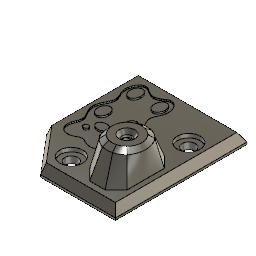
filament_sensor_cover_pc4-m10 (Autodesk Fusion 360 archive; units mm, degrees)
design "filament_sensor_cover"
Autodesk Fusion 360 part; units mm, degrees
sketch "base" plane through (0, 0, 0) normal (0, 0, 1) x (1, 0, 0)
  line L0 (0, 0) -> (27.1, 0)
  line L1 (27.1, 0) -> (27.1, 33.5)
  line L2 (27.1, 33.5) -> (0, 33.5)
  line L3 (0, 33.5) -> (0, 0)
  circle A0 centre (22.25, 23.5) radius 1.65
  circle A1 centre (20.05, 10) radius 2.2
  circle A2 centre (10.4, 5.5) radius 1.65
  circle A3 centre (20.05, 10) radius 1.3
  circle A4 centre (20.05, 10) radius 4.75
  line L4 (0, 9.5936) -> (8.05, 0)
  line L5 (24.8, 14.75) -> (24.8, 5.25)
  line L6 (24.8, 5.25) -> (22.0175, 2.4675)
  line L7 (22.0175, 2.4675) -> (18.0825, 2.4675)
  line L8 (18.0825, 2.4675) -> (15.3, 5.25)
  line L9 (15.3, 5.25) -> (15.3, 14.75)
  line L10 (24.8, 14.75) -> (22.0175, 17.5325)
  line L11 (22.0175, 17.5325) -> (18.0825, 17.5325)
  line L12 (18.0825, 17.5325) -> (15.3, 14.75)
  circle A5 centre (10.4, 5.5) radius 2.9
  circle A6 centre (22.25, 23.5) radius 2.9
  dimension "d4" = 3.3
  dimension "d5" = 3.3
  dimension "d6" = 4.4
  dimension "d7" = 2.6
  dimension "d11" = 2.2
  dimension "d15" = 9.65
  dimension "d21" = 9.5
  dimension "d78" = 10
  dimension "d85" = 20.05
  dimension "d94" = 7.05
  dimension "d139" = 13.5
  dimension "d141" = 4.5
  dimension "d142" = 40
  dimension "d151" = 45
  dimension "d152" = 45
  dimension "d153" = 9.5
  dimension "d154" = 45
  dimension "d155" = 45
  dimension "d159" = 5.8
  dimension "d160" = 5.8
  dimension "d163" = 23.5
  dimension "d166" = 12
  measures "d4" diameter of A0
  measures "d5" diameter of A2
  measures "d6" diameter of A1
  measures "d7" diameter of A3
  measures "d11" distance of L0.start
  measures "d21" diameter of A4
  measures "d85" distance of L0.start
  measures "d139" distance of L0.start
  measures "d142" angle of L3 L4
  measures "d151" angle of L7 L8
  measures "d152" angle of L6 L7
  measures "d154" angle of L11 L12
  measures "d155" angle of L10 L11
  measures "d159" diameter of A5
  measures "d160" diameter of A6
extrude "Extrude1" add sketch "base" against normal blind 3 contours L0 L1 L2 L3 L4 | A4 L5 L6 L7 L8 L9 | A4 L5 L9 L10 L11 L12 | A5 | A6
extrude "Extrude3" add sketch "base" along normal blind 7.5 and the other way up to surface (3 mm away) contours A1 | A3 | A4
loft "Loft1" add profiles "base" section 1 contours A1 | A3 | A4 | A4 L5 L6 L7 L8 L9 | A4 L5 L9 L10 L11 L12 section 2 face at (21.2351, 11.0499, 7.5)
extrude "Extrude12" cut sketch "base" along normal mid plane 20 contours A1 | A3
extrude "Extrude4" add sketch "base" against normal blind 2 from surface at 7.5 contours A1
extrude "Extrude16" cut sketch "base" against normal blind 1 contours A5 | A6
chamfer "Chamfer1" distance 1 angle 45 8 edges at (20.05, 5.25, 7.5) (17.688, 5.8789, 7.5) (24.8, 10, 7.5) (22.4315, 14.1099, 7.5) (20.0725, 14.7499, 7.5) (17.688, 14.1211, 7.5) (15.3, 10, 7.5) (22.412, 5.8789, 7.5)
chamfer "Chamfer2" distance 1 distance2 0.7 1 edges at (18.838, 9.5299, 7.5) measured on face at (21.3435, 9.8706, 6.8333)
chamfer "Chamfer4" distance 1 distance2 2.4 4 edges at (4.025, 4.7968, 0) (0, 21.5468, 0) (27.1, 16.75, 0) (17.575, 0, 0) measured on face at (5.1, 19.2812, 0) measured on face at (5.1, 19.2812, 0) measured on face at (5.1, 19.2812, 0) measured on face at (5.1, 19.2812, 0)
chamfer "Chamfer15" distance 1.6 distance2 2.4 1 edges at (13.55, 33.5, 0) measured on face at (5.7667, 19.4025, 0)
chamfer "Chamfer22" distance 0.3 angle 45 2 edges at (8.8617, 4.9033, -3) (20.7117, 22.9033, -3)
sketch "in_air_hole" plane through (0, 0, 5.5) normal (0, 0, -1) x (1, 0, 0)
  line L0 (18.2752, -8.7) -> (21.8248, -8.7)
  line L1 (18.2752, -11.3) -> (21.8248, -11.3)
  line L2 (21.35, -8.7) -> (21.35, -11.3)
  line L3 (18.75, -8.7) -> (18.75, -11.3)
  circle A0 centre (20.05, -10) radius 1.3
  circle A1 centre (20.05, -10) radius 2.2
extrude "Extrude10" cut sketch "in_air_hole" against normal blind 0.2 contours L0 L1 L3 A1 | L0 L1 L2 A1
extrude "Extrude11" cut sketch "in_air_hole" against normal blind 0.4 contours L0 L3 A0 | L0 L2 A0 | L1 L3 A0 | L1 L2 A0
sketch "Sketch12" plane through (0, 0, -3) normal (0, 0, -1) x (1, 0, 0)
  circle A0 centre (20.05, -10) radius 2.2
  line L0 (8.05, 0) -> (0, -9.5936)
  line L1 (0, -9.5936) -> (0, -33.5)
  line L2 (0, -33.5) -> (27.1, -33.5)
  line L3 (27.1, -33.5) -> (27.1, 0)
  line L4 (27.1, 0) -> (8.05, 0)
  circle A1 centre (20.05, -10) radius 2.2
  line L5 (0, -33.5) -> (27.1, -33.5)
  line L6 (23.85, -2.4) -> (16.55, -2.4)
  line L7 (16.55, -2.4) -> (16.55, -18.3)
  line L8 (16.55, -18.3) -> (23.85, -18.3)
  line L9 (23.85, -18.3) -> (23.85, -2.4)
  line L10 (16.55, -7.5) -> (23.85, -7.5)
  line L11 (16.55, -12.5) -> (23.85, -12.5)
  line L12 (22.55, -7.5) -> (22.55, -12.5)
  line L13 (17.55, -7.5) -> (17.55, -12.5)
  line L14 (6.25, -8.7) -> (9.35, -8.7)
  line L15 (9.35, -8.7) -> (9.35, -26.3)
  line L16 (9.35, -26.3) -> (6.25, -26.3)
  line L17 (6.25, -26.3) -> (6.25, -8.7)
  circle A2 centre (20.05, -10) radius 2.5
  circle A3 centre (10.4, -5.5) radius 1.95
  dimension "d239" = 3.8
  dimension "d240" = 7.6
  dimension "d241" = 3.5
  dimension "d242" = 8.3
  dimension "d249" = 3.1
  dimension "d251" = 17.6
  dimension "d252" = 10.7
  dimension "d254" = 0.3
  dimension "d259" = 3.2
  measures "d239" distance of L9
  measures "d240" distance of L6
  measures "d241" distance of L7
  measures "d242" distance of L8
  measures "d249" distance of L15 L17
  measures "d252" distance of L15
  measures "d254" distance of A0 A2
  measures "d259" distance of L14
extrude "Extrude17" cut sketch "Sketch12" against normal blind 1.4 contours L6 L7 L9 L10 | L9 L10 L11 L12 | L7 L10 L11 L13 | L7 L8 L9 L11 | L10 L12 A2 | L10 L13 A2 | L11 L12 A2 | A2 | L11 L13 A2 | L14 L15 L16 L17
extrude "Extrude19" cut sketch "Sketch12" against normal blind 0.2 from surface at -1.4 contours L9 L10 L11 L12 | L7 L10 L11 L13
extrude "Extrude20" cut sketch "Sketch12" against normal blind 0.4 from surface at -1.4 contours A0 A1 | L10 L12 A2 | L10 L13 A2 | L11 L12 A2 | A2 | L11 L13 A2
extrude "Extrude21" cut sketch "Sketch12" against normal blind 0.5 draft -45 from surface at -1.8 contours A0 A1 | A2
chamfer "Chamfer21" distance 0.5 angle 45 5 edges at (6.25, 17.5, -3) (9.35, 17.5, -3) (7.8, 8.7, -3) (23.85, 10.35, -3) (20.2, 2.4, -3)
sketch "logo" plane through (0, 0, 0) normal (0, 0, 1) x (-1, 0, 0)
  line L0 (-7.6627, -29.107) -> (-7.9745, -29.1444)
  line L1 (-7.9745, -29.1444) -> (-8.3459, -29.2538)
  line L2 (-8.3459, -29.2538) -> (-8.7523, -29.427)
  line L3 (-8.7523, -29.427) -> (-9.1647, -29.6489)
  line L4 (-9.1647, -29.6489) -> (-9.5618, -29.8965)
  line L5 (-9.5618, -29.8965) -> (-9.9376, -30.1385)
  line L6 (-9.9376, -30.1385) -> (-10.3005, -30.3388)
  line L7 (-10.3005, -30.3388) -> (-10.6648, -30.4618)
  line L8 (-10.6648, -30.4618) -> (-11.0429, -30.4781)
  line L9 (-11.0429, -30.4781) -> (-11.4365, -30.37)
  line L10 (-11.4365, -30.37) -> (-11.834, -30.1332)
  line L11 (-11.834, -30.1332) -> (-12.214, -29.7753)
  line L12 (-12.214, -29.7753) -> (-12.5496, -29.3123)
  line L13 (-12.5496, -29.3123) -> (-12.8133, -28.7661)
  line L14 (-12.8133, -28.7661) -> (-12.9814, -28.1613)
  line L15 (-12.9814, -28.1613) -> (-13.0387, -27.5233)
  line L16 (-13.0387, -27.5233) -> (-12.9808, -26.8757)
  line L17 (-12.9808, -26.8757) -> (-12.8192, -26.2395)
  line L18 (-12.8192, -26.2395) -> (-12.5836, -25.6303)
  line L19 (-12.5836, -25.6303) -> (-12.3262, -25.0573)
  line L20 (-12.3262, -25.0573) -> (-12.1178, -24.521)
  line L21 (-12.1178, -24.521) -> (-12.0118, -24.0146)
  line L22 (-12.0118, -24.0146) -> (-12.0257, -23.526)
  line L23 (-12.0257, -23.526) -> (-12.1502, -23.042)
  line L24 (-12.1502, -23.042) -> (-12.358, -22.5502)
  line L25 (-12.358, -22.5502) -> (-12.6136, -22.0431)
  line L26 (-12.6136, -22.0431) -> (-12.8804, -21.5194)
  line L27 (-12.8804, -21.5194) -> (-13.1248, -20.9829)
  line L28 (-13.1248, -20.9829) -> (-13.318, -20.4413)
  line L29 (-13.318, -20.4413) -> (-13.438, -19.9032)
  line L30 (-13.438, -19.9032) -> (-13.4715, -19.3767)
  line L31 (-13.4715, -19.3767) -> (-13.4161, -18.8673)
  line L32 (-13.4161, -18.8673) -> (-13.2803, -18.3767)
  line L33 (-13.2803, -18.3767) -> (-13.0813, -17.9044)
  line L34 (-13.0813, -17.9044) -> (-12.8431, -17.4481)
  line L35 (-12.8431, -17.4481) -> (-12.593, -17.005)
  line L36 (-12.593, -17.005) -> (-12.36, -16.5737)
  line L37 (-12.36, -16.5737) -> (-12.1707, -16.1535)
  line L38 (-12.1707, -16.1535) -> (-12.048, -15.7441)
  line L39 (-12.048, -15.7441) -> (-12.0061, -15.3438)
  line L40 (-12.0061, -15.3438) -> (-12.0482, -14.948)
  line L41 (-12.0482, -14.948) -> (-12.1635, -14.5478)
  line L42 (-12.1635, -14.5478) -> (-12.328, -14.1315)
  line L43 (-12.328, -14.1315) -> (-12.5094, -13.6882)
  line L44 (-12.5094, -13.6882) -> (-12.6717, -13.2115)
  line L45 (-12.6717, -13.2115) -> (-12.7802, -12.7035)
  line L46 (-12.7802, -12.7035) -> (-12.8062, -12.1779)
  line L47 (-12.8062, -12.1779) -> (-12.7291, -11.6578)
  line L48 (-12.7291, -11.6578) -> (-12.5377, -11.1715)
  line L49 (-12.5377, -11.1715) -> (-12.2318, -10.7487)
  line L50 (-12.2318, -10.7487) -> (-11.8228, -10.4149)
  line L51 (-11.8228, -10.4149) -> (-11.3348, -10.1886)
  line L52 (-11.3348, -10.1886) -> (-10.8008, -10.0778)
  line L53 (-10.8008, -10.0778) -> (-10.2568, -10.0804)
  line L54 (-10.2568, -10.0804) -> (-9.7352, -10.1825)
  line L55 (-9.7352, -10.1825) -> (-9.2581, -10.3582)
  line L56 (-9.2581, -10.3582) -> (-8.8319, -10.5692)
  line L57 (-8.8319, -10.5692) -> (-8.4472, -10.7692)
  line L58 (-8.4472, -10.7692) -> (-8.087, -10.9124)
  line L59 (-8.087, -10.9124) -> (-7.7345, -10.9646)
  line L60 (-7.6627, -29.107) -> (-7.3505, -29.1419)
  line L61 (-7.3505, -29.1419) -> (-6.9782, -29.2483)
  line L62 (-6.9782, -29.2483) -> (-6.5705, -29.4184)
  line L63 (-6.5705, -29.4184) -> (-6.1563, -29.637)
  line L64 (-6.1563, -29.637) -> (-5.7572, -29.8814)
  line L65 (-5.7572, -29.8814) -> (-5.3795, -30.1203)
  line L66 (-5.3795, -30.1203) -> (-5.0151, -30.3179)
  line L67 (-5.0151, -30.3179) -> (-4.6498, -30.4379)
  line L68 (-4.6498, -30.4379) -> (-4.2717, -30.4513)
  line L69 (-4.2717, -30.4513) -> (-3.8789, -30.34)
  line L70 (-3.8789, -30.34) -> (-3.4832, -30.1001)
  line L71 (-3.4832, -30.1001) -> (-3.1061, -29.7391)
  line L72 (-3.1061, -29.7391) -> (-2.7742, -29.2735)
  line L73 (-2.7742, -29.2735) -> (-2.5149, -28.7253)
  line L74 (-2.5149, -28.7253) -> (-2.3514, -28.1192)
  line L75 (-2.3514, -28.1192) -> (-2.2993, -27.4807)
  line L76 (-2.2993, -27.4807) -> (-2.3622, -26.8337)
  line L77 (-2.3622, -26.8337) -> (-2.5289, -26.1987)
  line L78 (-2.5289, -26.1987) -> (-2.7694, -25.5914)
  line L79 (-2.7694, -25.5914) -> (-3.0314, -25.0205)
  line L80 (-3.0314, -25.0205) -> (-3.2439, -24.4858)
  line L81 (-3.2439, -24.4858) -> (-3.354, -23.9804)
  line L82 (-3.354, -23.9804) -> (-3.3439, -23.4917)
  line L83 (-3.3439, -23.4917) -> (-3.2232, -23.0066)
  line L84 (-3.2232, -23.0066) -> (-3.0193, -22.5132)
  line L85 (-3.0193, -22.5132) -> (-2.7677, -22.0041)
  line L86 (-2.7677, -22.0041) -> (-2.5051, -21.4782)
  line L87 (-2.5051, -21.4782) -> (-2.265, -20.9399)
  line L88 (-2.265, -20.9399) -> (-2.0761, -20.3967)
  line L89 (-2.0761, -20.3967) -> (-1.9605, -19.8577)
  line L90 (-1.9605, -19.8577) -> (-1.931, -19.331)
  line L91 (-1.931, -19.331) -> (-1.9905, -18.822)
  line L92 (-1.9905, -18.822) -> (-2.1302, -18.3326)
  line L93 (-2.1302, -18.3326) -> (-2.3329, -17.8618)
  line L94 (-2.3329, -17.8618) -> (-2.5748, -17.4073)
  line L95 (-2.5748, -17.4073) -> (-2.8283, -16.9663)
  line L96 (-2.8283, -16.9663) -> (-3.0649, -16.5368)
  line L97 (-3.0649, -16.5368) -> (-3.2574, -16.1182)
  line L98 (-3.2574, -16.1182) -> (-3.3834, -15.7097)
  line L99 (-3.3834, -15.7097) -> (-3.4284, -15.3098)
  line L100 (-3.4284, -15.3098) -> (-3.3894, -14.9137)
  line L101 (-3.3894, -14.9137) -> (-3.2774, -14.5126)
  line L102 (-3.2774, -14.5126) -> (-3.1162, -14.095)
  line L103 (-3.1162, -14.095) -> (-2.9383, -13.6502)
  line L104 (-2.9383, -13.6502) -> (-2.7798, -13.1722)
  line L105 (-2.7798, -13.1722) -> (-2.6752, -12.6635)
  line L106 (-2.6752, -12.6635) -> (-2.6535, -12.1377)
  line L107 (-2.6535, -12.1377) -> (-2.7347, -11.6182)
  line L108 (-2.7347, -11.6182) -> (-2.9299, -11.1335)
  line L109 (-2.9299, -11.1335) -> (-3.2391, -10.713)
  line L110 (-3.2391, -10.713) -> (-3.6508, -10.3826)
  line L111 (-3.6508, -10.3826) -> (-4.1406, -10.16)
  line L112 (-4.1406, -10.16) -> (-4.6754, -10.0536)
  line L113 (-4.6754, -10.0536) -> (-5.2193, -10.0605)
  line L114 (-5.2193, -10.0605) -> (-5.7401, -10.1666)
  line L115 (-5.7401, -10.1666) -> (-6.2158, -10.3461)
  line L116 (-6.2158, -10.3461) -> (-6.6403, -10.5606)
  line L117 (-6.6403, -10.5606) -> (-7.0233, -10.7635)
  line L118 (-7.0233, -10.7635) -> (-7.3825, -10.9096)
  line L119 (-7.3825, -10.9096) -> (-7.7345, -10.9646)
  spline S0 degree 3 poles (-10.5113, -14.067) (-10.5113, -14.4192) (-10.2258, -14.7048) (-9.8736, -14.7048) knots 0 0 0 0 1 1 1 1
  spline S1 degree 3 poles (-9.8736, -14.7048) (-9.5214, -14.7048) (-9.2359, -14.4192) (-9.2359, -14.067) knots 0 0 0 0 1 1 1 1
  spline S2 degree 3 poles (-9.2359, -14.067) (-9.2359, -13.7148) (-9.5214, -13.4293) (-9.8736, -13.4293) knots 0 0 0 0 1 1 1 1
  spline S3 degree 3 poles (-9.8736, -13.4293) (-10.2258, -13.4293) (-10.5113, -13.7149) (-10.5113, -14.067) knots 0 0 0 0 1 1 1 1
  spline S4 degree 3 poles (-6.1545, -16.0271) (-6.157, -15.399) (-6.8574, -14.8925) (-7.719, -14.8959) knots 0 0 0 0 1 1 1 1
  spline S5 degree 3 poles (-7.719, -14.8959) (-8.5805, -14.8993) (-9.2769, -15.4113) (-9.2744, -16.0395) knots 0 0 0 0 1 1 1 1
  spline S6 degree 3 poles (-9.2744, -16.0395) (-9.272, -16.6676) (-8.5715, -17.174) (-7.71, -17.1707) knots 0 0 0 0 1 1 1 1
  spline S7 degree 3 poles (-7.71, -17.1707) (-6.8484, -17.1672) (-6.1521, -16.6552) (-6.1545, -16.0271) knots 0 0 0 0 1 1 1 1
  spline S8 degree 3 poles (-6.2087, -14.05) (-6.2087, -14.4022) (-5.9231, -14.6877) (-5.5709, -14.6877) knots 0 0 0 0 1 1 1 1
  spline S9 degree 3 poles (-5.5709, -14.6877) (-5.2188, -14.6877) (-4.9332, -14.4022) (-4.9332, -14.05) knots 0 0 0 0 1 1 1 1
  spline S10 degree 3 poles (-4.9332, -14.05) (-4.9332, -13.6977) (-5.2188, -13.4123) (-5.5709, -13.4123) knots 0 0 0 0 1 1 1 1
  spline S11 degree 3 poles (-5.5709, -13.4123) (-5.9231, -13.4123) (-6.2087, -13.6977) (-6.2087, -14.05) knots 0 0 0 0 1 1 1 1
  spline S12 degree 3 poles (-11.0392, -21.4868) (-10.2826, -21.4868) (-9.6693, -20.6818) (-9.6693, -19.6888) knots 0 0 0 0 1 1 1 1
  spline S13 degree 3 poles (-9.6693, -19.6888) (-9.6693, -18.6958) (-10.2826, -17.8907) (-11.0392, -17.8907) knots 0 0 0 0 1 1 1 1
  spline S14 degree 3 poles (-11.0392, -17.8907) (-11.7957, -17.8907) (-12.4091, -18.6957) (-12.4091, -19.6888) knots 0 0 0 0 1 1 1 1
  spline S15 degree 3 poles (-12.4091, -19.6888) (-12.4091, -20.6818) (-11.7957, -21.4868) (-11.0392, -21.4868) knots 0 0 0 0 1 1 1 1
  spline S16 degree 3 poles (-4.3466, -21.4603) (-3.5901, -21.4543) (-2.9831, -20.6445) (-2.991, -19.6515) knots 0 0 0 0 1 1 1 1
  spline S17 degree 3 poles (-2.991, -19.6515) (-2.9988, -18.6585) (-3.6185, -17.8584) (-4.3752, -17.8644) knots 0 0 0 0 1 1 1 1
  spline S18 degree 3 poles (-4.3752, -17.8644) (-5.1317, -17.8703) (-5.7386, -18.6802) (-5.7308, -19.6731) knots 0 0 0 0 1 1 1 1
  spline S19 degree 3 poles (-5.7308, -19.6731) (-5.7229, -20.6662) (-5.1032, -21.4662) (-4.3466, -21.4603) knots 0 0 0 0 1 1 1 1
  spline S20 degree 3 poles (-10.745, -29.4495) (-9.9884, -29.4495) (-9.375, -28.6445) (-9.375, -27.6514) knots 0 0 0 0 1 1 1 1
  spline S21 degree 3 poles (-9.375, -27.6514) (-9.375, -26.6585) (-9.9883, -25.8534) (-10.745, -25.8534) knots 0 0 0 0 1 1 1 1
  spline S22 degree 3 poles (-10.745, -25.8534) (-11.5016, -25.8534) (-12.1149, -26.6585) (-12.1149, -27.6514) knots 0 0 0 0 1 1 1 1
  spline S23 degree 3 poles (-12.1149, -27.6514) (-12.1149, -28.6445) (-11.5015, -29.4495) (-10.745, -29.4495) knots 0 0 0 0 1 1 1 1
  spline S24 degree 3 poles (-4.5777, -29.425) (-3.8211, -29.419) (-3.2141, -28.6092) (-3.222, -27.6162) knots 0 0 0 0 1 1 1 1
  spline S25 degree 3 poles (-3.222, -27.6162) (-3.2299, -26.6232) (-3.8496, -25.8231) (-4.6062, -25.8292) knots 0 0 0 0 1 1 1 1
  spline S26 degree 3 poles (-4.6062, -25.8292) (-5.3628, -25.8352) (-5.9697, -26.645) (-5.9618, -27.638) knots 0 0 0 0 1 1 1 1
  spline S27 degree 3 poles (-5.9618, -27.638) (-5.9539, -28.6309) (-5.3343, -29.431) (-4.5777, -29.425) knots 0 0 0 0 1 1 1 1
extrude "Extrude9" cut sketch "logo" against normal blind 0.4
equation "m3_holes = 3.3 mm"
equation "d4 = m3_holes"
equation "d5 = m3_holes"
equation "m3_head = 6 mm"
equation "d22 = 13 mm - 4.5 mm - 3 mm + 2 mm"
equation "layer_height = 0.2 mm"
equation "d64 = -layer_height * 2"
equation "center_extruder_to_motor_screw = 11.25 mm"
equation "d139 = 8 mm + 5.5 mm"
equation "d152 = d151"
equation "d153 = d21"
equation "d155 = d154"
equation "d159 = m3_head - 0.2 mm"
equation "d160 = m3_head - 0.2 mm"
equation "extrusion_width = 0.45 mm"
equation "num_perimeters = 4"
equation "num_top_bottoms = 5"
equation "perimeters_thickness = num_perimeters * ( extrusion_width - 0.05 mm )"
equation "top_bottom_thickness = layer_height * num_top_bottoms"
equation "light_leak_clearance = 0.3 mm"
equation "d239 = 3.5 mm + light_leak_clearance"
equation "d240 = 7.3 mm + light_leak_clearance"
equation "d242 = 8 mm + light_leak_clearance"
equation "d244 = -layer_height"
equation "d247 = -layer_height * 2"
equation "d249 = 2.5 mm + light_leak_clearance * 2"
equation "d251 = 17 mm + light_leak_clearance * 2"
equation "d252 = 11 mm - light_leak_clearance"
equation "d259 = 3.5 mm - light_leak_clearance"
